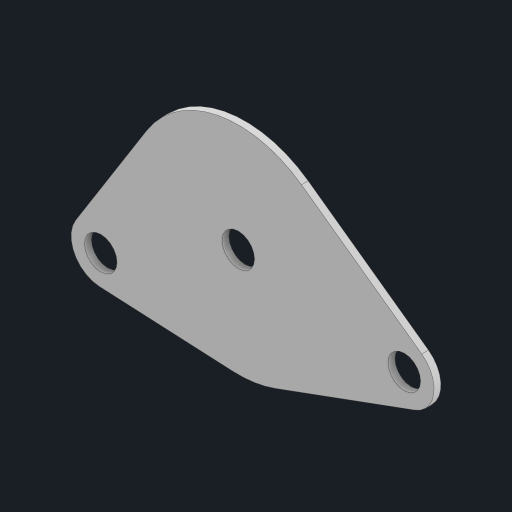
# Autodesk Inventor part: puncher gearbox
Saved by Autodesk Inventor 2023 (Build 270158000, 158)
## iProperties
Created: 2023-06-24
Part Number: puncher gearbox
Material: Generic
Document SubType Name: Modeling
Designer: reima
Density: 1 g/cm^3
Appearance: Default
Author: reima
Autodesk Inventor part; units mm, degrees
ref_plane "YZ Plane" through (0, 0, 0) normal (1, 0, 0) x (0, 1, 0)
ref_plane "XZ Plane" through (0, 0, 0) normal (0, 1, 0) x (-1, 0, 0)
ref_plane "XY Plane" through (0, 0, 0) normal (0, 0, 1) x (1, 0, 0)
sketch "Sketch1" plane through (0, 0, 0) normal (0, 0, 1) x (1, 0, 0)
  circle A0 centre (14.856, 3.7489) radius 2.032 projected
  circle A1 centre (53.8605, -1.6033) radius 3.81
  circle A2 centre (14.856, 3.7489) radius 3.81
  circle A3 centre (53.8605, -1.6033) radius 6.985
  arc A4 (29.6784, 24.3755) -> (23.5744, -20.108) centre (14.856, 3.7489) ccw
  line L0 (57.9367, 4.069) -> (29.6784, 24.3755)
  line L1 (23.5744, -20.108) -> (56.2581, -8.164)
  circle A5 centre (-17.4449, -13.0762) radius 3.81
  circle A6 centre (-17.4449, -13.0762) radius 6.985
  line L2 (-17.7932, -20.0525) -> (13.5893, -21.6195)
  line L3 (-23.3612, -9.3631) -> (-6.6579, 17.2512)
  point P0 (0, 0)
  dimension "d2" = 7.62
  dimension "d3" = 7.62
  dimension "d4" = 39.37
  dimension "d5" = 13.97
  dimension "d6" = 50.8
  dimension "d7" = 7.62
  dimension "d8" = 13.97
  constraints: 8 end point, 8 point on circle, 8 tangent, 6 centre point, 4 coincident
  measures "d2" diameter of A1
  measures "d3" diameter of A2
  measures "d4" distance of A0.centre A1.centre
  measures "d5" diameter of A3
  measures "d6" diameter of A4
  measures "d7" diameter of A5
  measures "d8" diameter of A6
extrude "Extrusion1" add sketch "Sketch1" along normal blind 1.5875 contours A3 | A3 L1 A4 L0 | A4 L2 A6 L3 | A6
body "Solid1"
